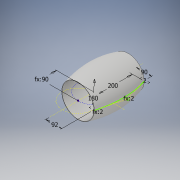
# Autodesk Inventor part: Form
Saved by Autodesk Inventor 2018.3 (Build 223284000, 284)
## iProperties
Created: 2018-07-22
Part Number: Form
Material: Generisch
Document SubType Name: Modeling
Designer: JochenAlt
Density: 1 g/cm^3
Appearance: Vorgabe
Author: JochenAlt
Autodesk Inventor part; units mm, degrees
ref_plane "YZ Plane" through (0, 0, 0) normal (1, 0, 0) x (0, 1, 0)
ref_plane "XZ Plane" through (0, 0, 0) normal (0, 1, 0) x (-1, 0, 0)
ref_plane "XY Plane" through (0, 0, 0) normal (0, 0, 1) x (1, 0, 0)
sketch "Skizze3" plane through (0, 0, 0) normal (0, 0, 1) x (1, 0, 0)
  line L0 (0, 279.5849) -> (0, -256.3854) construction
  line L1 (-135.3027, 0) -> (181.8164, 0) construction
  line L2 (92, 200) -> (90, 200)
  circle A0 centre (0, 0) radius 90 construction
  circle A1 centre (0, -90) radius 89.8182 construction
  line L3 (92, -90) -> (94, -90)
  line L4 (92, -90) -> (131.3459, 65.056) construction
  line L5 (131.3459, 65.056) -> (90, 200) construction
  spline S0 degree 2 poles (92, -90) (131.3459, 65.056) (90, 200) knots 1 1 1 2 2 2
  line L6 (92, 200) -> (136.5137, 65.056) construction
  line L7 (136.5137, 65.056) -> (94, -90) construction
  spline S1 degree 2 poles (92, 200) (136.5137, 65.056) (94, -90) knots 1 1 1 2 2 2
  line L8 (131.3459, 65.056) -> (133.3459, 65.056) construction
  point P0 (90, 149.8145)
  dimension "d7" = 200
  dimension "d11" = 2
  dimension "d12" = 92
  dimension "d13" = 180
  dimension "d14" = 90
  dimension "d15" = 90
  dimension "d18" = 2
  dimension "d19" = 2
  constraints: 6 end point, 3 horizontal, 2 centre point, 2 coincident, 2 point on line, 6 other
  measures "d7" distance between parallel lines of L1 L2
  measures "d11" distance of L2.start L2.end
  measures "d12" distance from line of L0 L3.start
  measures "d13" diameter of A0
  measures "d14" distance of A1.centre point (0, 0)
  measures "d15" distance from line of L0 L2.end
  measures "d18" distance of L3.end L3.start
  measures "d19" distance of L8.start L8.end
revolve "Umdrehung1" add sketch "Skizze3" angle 360 about axis through (0, 0, 0) along (0, -1, 0)
equation "\"d14\" = 0.5 * d13"
equation "\"d18\" = d17"
equation "\"d16\" = d11"
equation "\"d17\" = d16"
